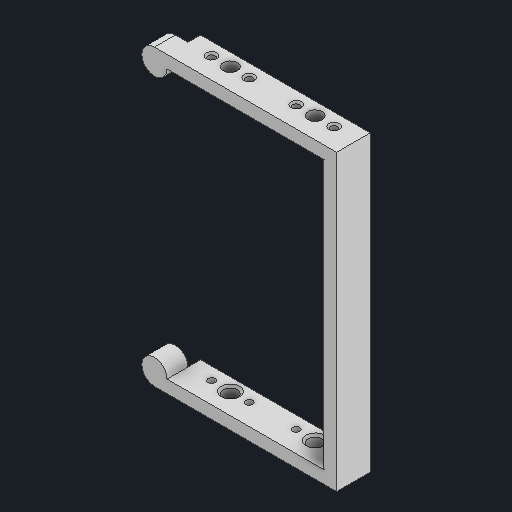
# Autodesk Inventor part: bmw2
Saved by Autodesk Inventor 2026.2 (Build 302298010, 298A)
## iProperties
Created: 2026-09-07
Part Number: bmw2
Material: Generic
Document SubType Name: Modeling
Designer: karol
Density: 1 g/cm^3
Appearance: Default
Author: karol
Autodesk Inventor part; units mm, degrees
ref_plane "YZ Plane" through (0, 0, 0) normal (1, 0, 0) x (0, 1, 0)
ref_plane "XZ Plane" through (0, 0, 0) normal (0, 1, 0) x (-1, 0, 0)
ref_plane "XY Plane" through (0, 0, 0) normal (0, 0, 1) x (1, 0, 0)
sketch "Sketch1" plane through (0, 0, 0) normal (0, 0, 1) x (1, 0, 0)
  line L0 (-58, -60) -> (-60, -60) projected
  line L1 (-60, -60) -> (-60, -39.5) projected
  line L2 (-60, -39.5) -> (-58, -39.5) projected
  line L3 (-58, -39.5) -> (-58, -60) projected
  line L4 (49.6, 30) -> (51.6, 30) projected
  line L5 (51.6, 30) -> (51.6, 9.5) projected
  line L6 (51.6, 9.5) -> (49.6, 9.5) projected
  line L7 (49.6, 9.5) -> (49.6, 30) projected
  line L8 (-58, 39.5) -> (-60, 39.5) projected
  line L9 (-60, 39.5) -> (-60, 60) projected
  line L10 (-60, 60) -> (-58, 60) projected
  line L11 (-58, 60) -> (-58, 39.5) projected
  line L12 (-21.6, -39.5) -> (-19.6, -39.5) projected
  line L13 (-19.6, -39.5) -> (-19.6, -60) projected
  line L14 (-19.6, -60) -> (-21.6, -60) projected
  line L15 (-21.6, -60) -> (-21.6, -39.5) projected
  line L16 (51.6, -30) -> (49.6, -30) projected
  line L17 (49.6, -30) -> (49.6, -9.5) projected
  line L18 (49.6, -9.5) -> (51.6, -9.5) projected
  line L19 (51.6, -9.5) -> (51.6, -30) projected
  line L20 (-21.6, 60) -> (-19.6, 60) projected
  line L21 (-19.6, 60) -> (-19.6, 39.5) projected
  line L22 (-19.6, 39.5) -> (-21.6, 39.5) projected
  line L23 (-21.6, 39.5) -> (-21.6, 60) projected
  line L24 (90, -35) -> (90, 35) projected
  line L25 (90, 35) -> (49.6, 35) projected
  line L26 (49.6, 35) -> (49.6, 60) projected
  line L27 (49.6, 60) -> (90, 60) projected
  line L28 (90, 60) -> (90, 90) projected
  line L29 (90, 90) -> (-19.6, 90) projected
  line L30 (-19.6, 90) -> (-19.6, 65) projected
  line L31 (-19.6, 65) -> (-60, 65) projected
  line L32 (-60, 65) -> (-60, 90) projected
  line L33 (-60, 90) -> (-90, 90) projected
  line L34 (-90, 90) -> (-90, -90) projected
  line L35 (-90, -90) -> (-60, -90) projected
  line L36 (-60, -90) -> (-60, -65) projected
  line L37 (-60, -65) -> (-19.6, -65) projected
  line L38 (-19.6, -65) -> (-19.6, -90) projected
  line L39 (-19.6, -90) -> (90, -90) projected
  line L40 (90, -90) -> (90, -60) projected
  line L41 (90, -60) -> (49.6, -60) projected
  line L42 (49.6, -60) -> (49.6, -35) projected
  line L43 (49.6, -35) -> (90, -35) projected
  line L44 (86, -32) -> (73.8, -32) projected
  line L45 (73.8, -32) -> (73.8, -7.5) projected
  line L46 (73.8, -7.5) -> (86, -7.5) projected
  line L47 (86, -7.5) -> (86, -32) projected
  line L48 (65.8, -32) -> (53.6, -32) projected
  line L49 (53.6, -32) -> (53.6, -7.5) projected
  line L50 (53.6, -7.5) -> (65.8, -7.5) projected
  line L51 (65.8, -7.5) -> (65.8, -32) projected
  line L52 (86, -86) -> (70.6, -86) projected
  line L53 (70.6, -86) -> (70.6, -69.8) projected
  line L54 (70.6, -69.8) -> (86, -69.8) projected
  line L55 (86, -69.8) -> (86, -86) projected
  line L56 (86, 86) -> (86, 69.8) projected
  line L57 (86, 69.8) -> (70.6, 69.8) projected
  line L58 (70.6, 69.8) -> (70.6, 86) projected
  line L59 (70.6, 86) -> (86, 86) projected
  line L60 (73.8, 32) -> (86, 32) projected
  line L61 (86, 32) -> (86, 7.5) projected
  line L62 (86, 7.5) -> (73.8, 7.5) projected
  line L63 (73.8, 7.5) -> (73.8, 32) projected
  line L64 (65.8, 32) -> (65.8, 7.5) projected
  line L65 (65.8, 7.5) -> (53.6, 7.5) projected
  line L66 (53.6, 7.5) -> (53.6, 32) projected
  line L67 (53.6, 32) -> (65.8, 32) projected
  line L68 (-69.6, -87) -> (-85, -87) projected
  line L69 (-85, -87) -> (-85, -70.8) projected
  line L70 (-85, -70.8) -> (-69.6, -70.8) projected
  line L71 (-69.6, -70.8) -> (-69.6, -87) projected
  line L72 (-56, -62) -> (-56, -37.5) projected
  line L73 (-56, -37.5) -> (-43.8, -37.5) projected
  line L74 (-43.8, -37.5) -> (-43.8, -62) projected
  line L75 (-43.8, -62) -> (-56, -62) projected
  line L76 (-56, 62) -> (-43.8, 62) projected
  line L77 (-43.8, 62) -> (-43.8, 37.5) projected
  line L78 (-43.8, 37.5) -> (-56, 37.5) projected
  line L79 (-56, 37.5) -> (-56, 62) projected
  line L80 (-23.6, 62) -> (-23.6, 37.5) projected
  line L81 (-23.6, 37.5) -> (-35.8, 37.5) projected
  line L82 (-35.8, 37.5) -> (-35.8, 62) projected
  line L83 (-35.8, 62) -> (-23.6, 62) projected
  line L84 (-23.6, -62) -> (-35.8, -62) projected
  line L85 (-35.8, -62) -> (-35.8, -37.5) projected
  line L86 (-35.8, -37.5) -> (-23.6, -37.5) projected
  line L87 (-23.6, -37.5) -> (-23.6, -62) projected
  line L88 (-85, 87) -> (-69.6, 87) projected
  line L89 (-69.6, 87) -> (-69.6, 70.8) projected
  line L90 (-69.6, 70.8) -> (-85, 70.8) projected
  line L91 (-85, 70.8) -> (-85, 87) projected
  line L92 (49.6, 35) -> (90, 35)
  line L93 (90, 35) -> (90, 32)
  line L94 (90, 32) -> (49.6, 32)
  line L95 (49.6, 32) -> (49.6, 35)
  line L96 (90, 35) -> (87, 35)
  line L97 (87, 35) -> (87, -35)
  line L98 (87, -35) -> (90, -35)
  line L99 (90, -35) -> (90, 35)
  line L100 (87, -35) -> (49.6, -35)
  line L101 (49.6, -35) -> (49.6, -32)
  line L102 (49.6, -32) -> (87, -32)
  line L103 (87, -32) -> (87, -35)
  circle A0 centre (-63, -65) radius 1.5 projected
  circle A1 centre (-16.6, -87) radius 1.5 projected
  circle A2 centre (49.6, -87) radius 1.5 projected
  circle A3 centre (46.6, -60) radius 1.5 projected
  circle A4 centre (87, -63) radius 1.5 projected
  circle A5 centre (46.6, -32) radius 1.5 projected
  circle A6 centre (46.6, 32) radius 1.5 projected
  circle A7 centre (87, 63) radius 1.5 projected
  circle A8 centre (46.6, 60) radius 1.5 projected
  circle A9 centre (49.6, 87) radius 1.5 projected
  circle A10 centre (-16.6, 87) radius 1.5 projected
  circle A11 centre (-16.6, 65) radius 1.5 projected
  circle A12 centre (-63, 65) radius 1.5 projected
  line L104 (-76, -39.25) -> (-82, -39.25) projected
  line L105 (-82, -39.25) -> (-82, -20.75) projected
  line L106 (-82, -20.75) -> (-76, -20.75) projected
  line L107 (-76, -20.75) -> (-76, -39.25) projected
  line L108 (-76, 20.75) -> (-82, 20.75) projected
  line L109 (-82, 20.75) -> (-82, 39.25) projected
  line L110 (-82, 39.25) -> (-76, 39.25) projected
  line L111 (-76, 39.25) -> (-76, 20.75) projected
  circle A13 centre (-86.5, -55.7158) radius 1.25 projected
  circle A14 centre (-86.5, 55.8) radius 1.25 projected
  circle A15 centre (-79.5, -5.4579) radius 1.25 projected
  circle A16 centre (-79.5, 5.5421) radius 1.25 projected
  point P0 (0, 0)
  point P1 (87, 32)
  dimension "d0" = 3
  constraints: 24 end point, 6 parallel, 3 horizontal, 3 perpendicular, 2 point on line
  measures "d0" distance of L98.end L97.end
extrude "Extrusion1" add sketch "Sketch1" along normal blind 8 contours L43 L97 L94 L24 | L94 L97 L25 L24 | L43 L101 L102 L48 L44 L97 | L94 L60 L67 L95 L25 L97
sketch "Sketch2" plane through (49.6, -35, 0) normal (-1, 0, 0) x (0, 0, 1)
  line L0 (8, 0) -> (8, 70) projected
  line L1 (8, 70) -> (3, 70)
  line L2 (3, 70) -> (3, 64)
  line L3 (3, 64) -> (8, 64)
  line L4 (8, 64) -> (8, 70)
  line L5 (8, 0) -> (3, 0)
  line L6 (3, 0) -> (3, 6)
  line L7 (3, 6) -> (8, 6)
  line L8 (8, 6) -> (8, 0)
  point P0 (0, 35)
  dimension "d3" = 5
  dimension "d4" = 6
  dimension "d5" = 5
  dimension "d6" = 6
  constraints: 16 end point, 4 parallel, 2 horizontal, 2 perpendicular
  measures "d3" distance of L3.end L2.end
  measures "d4" distance of L2.end L1.end
  measures "d5" distance of L6.end L7.end
  measures "d6" distance of L5.end L6.end
extrude "Extrusion2" add sketch "Sketch2" along normal blind 6
sketch "Sketch3" plane through (49.6, 29, 3) normal (0, 0, -1) x (-1, 0, 0)
  line L0 (0, 0) -> (6, 0) projected
  line L1 (0, 6) -> (6, 6) projected
  line L2 (0, 0) -> (6, 6)
  line L3 (6, 6) -> (0, 6)
  line L4 (0, 6) -> (6, 0)
  circle A0 centre (3, 3) radius 2
  point P0 (49.6, -29)
  dimension "d9" = 4
  constraints: 6 end point, 1 centre point, 1 collinear, 1 midpoint, 1 perpendicular
  measures "d9" diameter of A0
extrude "Extrusion3" cut sketch "Sketch3" against normal blind 4 contours A0 L4 L2 | L2 L4 A0 | L4 L2 A0 | L4 A0 L2
sketch "Sketch4" plane through (49.6, -32, 3) normal (0, 0, -1) x (-1, 0, 0)
  line L0 (0, -3) -> (6, -3) projected
  line L1 (0, -3) -> (6, 3)
  line L2 (6, 3) -> (6, -3)
  line L3 (0, 3) -> (6, 3) projected
  line L4 (6, -3) -> (0, 3)
  circle A0 centre (3, 0) radius 2
  point P0 (49.6, 32)
  dimension "d12" = 4
  constraints: 6 end point, 1 centre point, 1 midpoint, 1 perpendicular
  measures "d12" diameter of A0
extrude "Extrusion4" cut sketch "Sketch4" against normal blind 4 contours A0 L4 L1 | L1 L4 A0 | L4 L1 A0 | L4 A0 L1
fillet "Fillet1" radius 3 6 edges at (49.6, -29, 5.5) (43.6, -29, 5.5) (43.6, 35, 5.5) (43.6, 29, 5.5) (43.6, -35, 5.5) (49.6, 29, 5.5)
sketch "Sketch5" plane through (49.6, 35, 0) normal (0, 1, 0) x (1, 0, 0)
  circle A0 centre (34.8, -3) radius 0.85
  circle A1 centre (30.3, -3) radius 1.7
  circle A2 centre (25.8, -3) radius 0.85
  circle A3 centre (14.6, -3) radius 0.85
  circle A4 centre (10.1, -3) radius 1.7
  circle A5 centre (5.6, -3) radius 0.85
  line L0 (40.4, 0) -> (0, 0) projected
  line L1 (40.4, 0) -> (40.4, -8) projected
  point P0 (-49.6, 0)
  point P1 (40.4, -4)
  dimension "d16" = 1.7
  dimension "d17" = 3.4
  dimension "d18" = 1.7
  dimension "d19" = 1.7
  dimension "d20" = 3.4
  dimension "d21" = 1.7
  dimension "d22" = 3
  dimension "d23" = 3
  dimension "d24" = 3
  dimension "d25" = 3
  dimension "d26" = 3
  dimension "d27" = 3
  dimension "d28" = 4.5
  dimension "d29" = 4.5
  dimension "d31" = 4.5
  dimension "d32" = 4.5
  dimension "d33" = 20.2
  dimension "d34" = 10.1
  constraints: 6 centre point, 1 midpoint
  measures "d16" diameter of A0
  measures "d17" diameter of A1
  measures "d18" diameter of A2
  measures "d19" diameter of A3
  measures "d20" diameter of A4
  measures "d21" diameter of A5
  measures "d22" distance from line of L0 A0.centre
  measures "d23" distance from line of L0 A1.centre
  measures "d24" distance from line of L0 A2.centre
  measures "d25" distance from line of L0 A3.centre
  measures "d26" distance from line of L0 A4.centre
  measures "d27" distance from line of L0 A5.centre
  measures "d28" distance of A1.centre A0.centre
  measures "d29" distance of A2.centre A1.centre
  measures "d31" distance of A4.centre A3.centre
  measures "d32" distance of A5.centre A4.centre
  measures "d33" distance of A1.centre A4.centre
  measures "d34" distance from line of L1 A1.centre
extrude "Extrusion5" cut sketch "Sketch5" against normal blind 3
sketch "Sketch6" plane through (49.6, -35, 0) normal (0, -1, 0) x (1, 0, 0)
  circle A0 centre (5.6, 3) radius 0.85 projected
  circle A1 centre (10.1, 3) radius 1.7 projected
  circle A2 centre (14.6, 3) radius 0.85 projected
  circle A3 centre (25.8, 3) radius 0.85 projected
  circle A4 centre (30.3, 3) radius 1.7 projected
  circle A5 centre (34.8, 3) radius 0.85 projected
  point P0 (-49.6, 0)
extrude "Extrusion6" cut sketch "Sketch6" against normal blind 3
fillet "Fillet2" radius 0.5 4 edges at (58, 32, 3) (78.2, 32, 3) (78.2, -32, 3) (58, -32, 3) inverted yes
chamfer "Chamfer1" distance 0.4 angle 45 8 edges at (83.55, 35, 3) (74.55, 35, 3) (63.35, 35, 3) (54.35, 35, 3) (63.35, -35, 3) (54.35, -35, 3) (74.55, -35, 3) (83.55, -35, 3)
body "Solid1"
